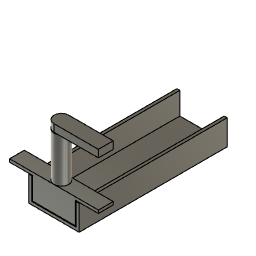
design (Autodesk Fusion 360 design; units mm, degrees)
Autodesk Fusion 360 part; units mm, degrees
sketch "Sketch1" plane through (0, 0, 0) normal (0, 1, 0) x (1, 0, 0)
  line L0 (0, 0) -> (150, 0)
  line L1 (150, 0) -> (150, -150)
  line L2 (150, -150) -> (170, -150)
  line L3 (170, -150) -> (170, 0)
  line L4 (170, 0) -> (150, 0) construction
  line L5 (150, 0) -> (150, 20) construction
  line L6 (150, 20) -> (0, 20)
  line L7 (0, 20) -> (0, 0)
  line L8 (150, 20) -> (170, 20)
  line L9 (170, 20) -> (170, 0)
  line L10 (0, -1.75) -> (0, -22.5)
  line L11 (-170, 0) -> (-150, 0) construction
  line L12 (0, 0) -> (-150, 0)
  line L13 (-150, 20) -> (-170, 20)
  line L14 (0, 20) -> (0, 0) construction
  line L15 (-170, -150) -> (-170, 0)
  line L16 (-150, -150) -> (-170, -150)
  line L17 (-150, 20) -> (0, 20)
  line L18 (-170, 20) -> (-170, 0)
  line L19 (-150, 0) -> (-150, -150)
  line L20 (-150, 0) -> (-150, 20) construction
  line L21 (150, 0) -> (145, 0)
  line L22 (145, 0) -> (145, -5)
  line L23 (145, -5) -> (150, -5)
  line L24 (150, -5) -> (150, 0)
  line L25 (150, 0) -> (145, 0)
  line L26 (145, 0) -> (145, -5)
  line L27 (145, -5) -> (0, -5)
  line L28 (0, -5) -> (0, 0)
  line L29 (150, -150) -> (145, -150)
  line L30 (145, -150) -> (145, -5)
  line L31 (0, -5) -> (145, -5)
  line L32 (145, -5) -> (145, -150)
  line L33 (145, -150) -> (0, -150)
  line L34 (0, -150) -> (0, -5)
  line L35 (145, -150) -> (145, -155)
  line L36 (145, -155) -> (0, -155)
  line L37 (0, -155) -> (0, -150)
  line L38 (0, -150) -> (145, -150)
  line L39 (145, -150) -> (145, -155)
  line L40 (0, -155) -> (300, -155)
  line L41 (300, -155) -> (300, -175)
  line L42 (0, -155) -> (300, -155)
  line L43 (300, -155) -> (300, -175)
  line L44 (300, -175) -> (0, -175)
  line L45 (0, -175) -> (0, -155)
  line L46 (-300, -155) -> (-300, -175)
  line L47 (-300, -175) -> (0, -175)
  line L48 (0, -175) -> (0, -155)
  line L49 (0, -155) -> (-300, -155)
  line L50 (-145, -150) -> (-145, -155)
  line L51 (-145, -150) -> (-145, -5)
  line L52 (0, -155) -> (0, -150)
  line L53 (0, -150) -> (0, -5)
  line L54 (-145, -5) -> (0, -5)
  constraint coincident L0.start L7.end
  constraint horizontal L0
  constraint perpendicular L0 L1
  constraint equal L0 L1
  constraint perpendicular L1 L2
  constraint perpendicular L0 L3
  constraint perpendicular L1 L4
  constraint perpendicular L4 L5
  constraint perpendicular L5 L6
  constraint perpendicular L6 L7
  constraint perpendicular L3 L8
  constraint perpendicular L4 L9
  constraint equal L8 L9
  constraint symmetric L0.start L10 L7.end
  constraint symmetric L0.end L10 L11.end
  constraint symmetric L1.end L10 L16.start
  constraint symmetric L2.end L10 L15.start
  constraint symmetric L3.end L10 L11.start
  constraint symmetric L5.end L10 L13.start
  constraint symmetric L6.end L10 L7.start
  constraint symmetric L8.end L10 L13.end
  constraint perpendicular L5 L21
  constraint perpendicular L21 L22
  constraint equal L21 L22
  constraint horizontal L23
  constraint vertical L24
  constraint horizontal L25
  constraint vertical L26
  constraint perpendicular L10 L27
  constraint perpendicular L27 L28
  constraint perpendicular L1 L29
  constraint perpendicular L29 L30
  constraint horizontal L31
  constraint vertical L32
  constraint horizontal L33
  constraint vertical L34
  constraint perpendicular L33 L35
  constraint equal L29 L35
  constraint horizontal L36
  constraint vertical L37
  constraint horizontal L38
  constraint vertical L39
  constraint perpendicular L39 L40
  constraint perpendicular L40 L41
  constraint equal L8 L41
  constraint horizontal L42
  constraint vertical L43
  constraint horizontal L44
  constraint vertical L45
  constraint symmetric L22.end L28 L51.end
  constraint symmetric L27.end L28 L31.start
  constraint symmetric L28 L29.end L50.start
  constraint symmetric L28 L33.end L34.start
  constraint symmetric L28 L35.end L50.end
  constraint symmetric L28 L36.end L37.start
  constraint symmetric L28 L40.end L46.start
  constraint symmetric L28 L41.end L46.end
  constraint symmetric L28 L44.end L45.start
extrude "Extrude1" add sketch "Sketch1" along normal blind 1000 contours L0 L1 L2 L3 L6 L7 L8 L9 L21 L24 L25 | L7 L12 L13 L15 L16 L17 L18 L19 makes body 1
extrude "Extrude2" add sketch "Sketch1" along normal blind 100 separate body contours L10 L27 L30 L31 L32 L33 L34 L38 L53 | L10 L34 L37 L49 L50 L51 L52 L53 L54 | L33 L35 L36 L37 L38 L39 L40 L42 L52 | L36 L40 L41 L42 L43 L44 L45 L48 | L45 L46 L47 L48 L49 makes body 2
sketch "Sketch2" plane through (0, 0, 175) normal (0, 0, 1) x (-1, 0, 0)
  line L0 (300, 0) -> (-300, 0)
  line L1 (-300, 0) -> (-300, -100)
  line L2 (-300, -100) -> (300, -100)
  line L3 (300, -100) -> (300, 0)
  line L4 (0, 0) -> (0, -100)
  circle A0 centre (0, -50) radius 50
  constraint coincident L4.start origin
  constraint midpoint L2 L4.end
  constraint midpoint L4 A0.centre
  constraint coincident L4.end A0
extrude "Extrude3" add sketch "Sketch2" along normal blind 300 contours L4 A0 | L4 A0 bodies 2
extrude "Extrude4" add 1 faces at (4.883, 62.4417, 475) along direction (0, 0, 1) blind 50 from surface at 5 on bodies 2 bodies 2 makes body 3
sketch "Sketch3" plane through (0, 0, 530) normal (0, 0, 1) x (-1, 0, 0)
  circle A0 centre (0, -50) radius 50
  line L0 (0, 0) -> (0, -100)
  constraint coincident L0.start origin
  constraint coincident A0 L0.end
  constraint vertical L0
extrude "Extrude5" cut sketch "Sketch3" against normal blind 50 contours A0 L0 picked at (-24.3667, -35.1594) bodies 3
extrude "Extrude6" add 1 faces at (0, 33.3333, 513.3333) along direction (1, 0, 0) blind 400 on bodies 3 bodies 3
extrude "Extrude7" cut 1 faces at (400, 33.3333, 513.3333) along direction (-1, 0, 0) up to surface (100 mm away) on bodies 3 bodies 3
copy_body "Body->Comp1" bodies 1 removing the originals makes body 4 in component "base"
copy_body "Body->Comp2" bodies 2 removing the originals makes body 5 in component "slider"
copy_body "Body->Comp3" bodies 3 removing the originals makes body 6 in component "rotor"
component "base" placed x (1, 0, 0) y (0, 1, 0) z (0, 0, 1) at (0, 0, 0)
component "slider" placed x (1, 0, 0) y (0, 1, 0) z (0, 0, 1) at (0, 0, 0)
component "rotor" placed x (1, 0, 0) y (0, 1, 0) z (0, 0, 1) at (0, 0, 0)
